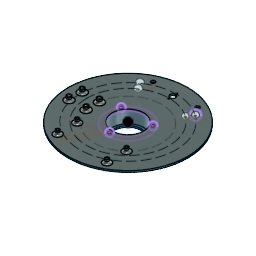
top_plate (Autodesk Fusion 360 design; units mm, degrees)
Autodesk Fusion 360 part; units mm, degrees
note: some values were not read from the file. Chosen so that the rebuilt part matches the saved one: which face or edge a step refers to. Set by a fixed rule: which sketch regions a step uses.
sketch "Sketch1" plane through (0, 0, 0) normal (0, 0, 1) x (1, 0, 0)
  circle A0 centre (0, 0) radius 80
  dimension "d1" = 160
  constraint coincident A0.centre origin
  measures "d1" diameter of A0
extrude "Extrude1" add sketch "Sketch1" along normal blind 2
sketch "Sketch4" plane through (0, 0, 2) normal (0, 0, 1) x (-1, 0, 0)
  circle A0 centre (0, 0) radius 80
  circle A1 centre (0, 0) radius 18
  dimension "d9" = 36
  constraint concentric A0 A1
  measures "d9" diameter of A1
extrude "Extrude3" cut sketch "Sketch4" against normal blind 20 contours A1 picked at (-10.335126, 0.653415)
sketch "Sketch5" plane through (0, 0, 2) normal (0, 0, 1) x (-1, 0, 0)
  circle A0 centre (0, 0) radius 18
  circle A1 centre (0, 0) radius 80
  circle A2 centre (0, 0) radius 21
  circle A3 centre (0, 0) radius 28
  dimension "d12" = 42
  dimension "d13" = 56
  constraint coincident A0.centre A1.centre
  constraint concentric A2 A3
  measures "d12" diameter of A2
  measures "d13" diameter of A3
extrude "Extrude4" add sketch "Sketch5" against normal blind 19 contours A3 picked at (25.562421, -1.391061)
sketch "Sketch6" plane through (0, 0, 2) normal (0, 0, -1) x (-1, 0, 0)
  circle A0 centre (0, 0) radius 21
  circle A1 centre (0, 0) radius 28
  circle A2 centre (0, -24.5) radius 2.15
  circle A3 centre (0, 0) radius 80
  circle A4 centre (0, 0) radius 18
  dimension "d118" = 4.3
  dimension "d119" = 24.5
  constraint vertical A0.centre A2.centre
  measures "d118" diameter of A2
  measures "d119" distance of A0.centre A2.centre
extrude "Extrude5" cut sketch "Sketch6" along normal blind 6.3 contours A2 picked at (0.840738, -23.965006)
pattern_circular "C-Pattern2" count 3 over 360 about axis through (0, 0, 2) along (0, 0, -1) of "Extrude5"
sketch "Sketch7" plane through (0, 0, 0) normal (0, 0, -1) x (1, 0, 0)
  circle A0 centre (0, 0) radius 18
  circle A1 centre (0, 0) radius 80
  circle A2 centre (0, 0) radius 45 construction
  circle A3 centre (0, 0) radius 21
  circle A4 centre (0, 0) radius 28
  dimension "d21" = 90
  constraint concentric A0 A2
  measures "d21" diameter of A2
sketch "Sketch8" plane through (0, 0, 0) normal (0, 0, -1) x (1, 0, 0)
  circle A0 centre (0, -60) radius 3.5
  circle A1 centre (0, -65.500001) radius 1
  circle A2 centre (0, -54.500001) radius 1
  dimension "d22" = 7
  dimension "d23" = 2
  dimension "d24" = 2
  measures "d22" diameter of A0
  measures "d23" diameter of A1
  measures "d24" diameter of A2
extrude "Extrude6" cut sketch "Sketch8" against normal blind 2
move_face "OffsetFaces1" offset -0.2 1 faces at (-20.895646, 2.090925, -5.666667)
ref_plane "WorkPlane1" through (0, 0, 12.125) normal (-0.819152, 0.573576, 0) x (0, 0, 1)
ref_plane "WorkPlane2" through (0, 0, 12.125) normal (-0.819152, -0.573576, 0) x (0, 0, 1)
sketch "Sketch9" plane through (0, 0, 2) normal (0, 0, 1) x (-1, 0, 0)
  circle A0 centre (0, 0) radius 80
  circle A1 centre (0, 0) radius 55 construction
  circle A2 centre (0, 0) radius 64.5 construction
  circle A3 centre (-21.217622, -12.25) radius 2.15
  circle A4 centre (21.217622, -12.25) radius 2.15
  circle A5 centre (0, 24.5) radius 2.15
  dimension "d31" = 110
  dimension "d32" = 129
  constraint coincident A0.centre A1.centre
  constraint concentric A0 A2
  measures "d31" diameter of A1
  measures "d32" diameter of A2
sketch "Sketch10" plane through (0, 0, 0) normal (-0.819152, -0.573576, 0) x (0, 0, 1)
  line L0 (2, 55.000001) -> (2, 64.500001) construction
  line L1 (2, 64.500001) -> (2, 65.000001)
  dimension "d34" = 9.5
  dimension "d43" = 0.5
  constraint vertical L0
  constraint parallel L0 L1
sketch "Sketch11" plane through (0, 0, 0) normal (-0.819152, 0.573576, 0) x (0, 0, 1)
  line L0 (2, 55.000001) -> (2, 64.500001) construction
  line L1 (2, 64.500001) -> (2, 65.000001) construction
  dimension "d36" = 9.5
  constraint vertical L0
  constraint parallel L0 L1
sketch "Sketch12" plane through (0, 0, 2) normal (0, 0, 1) x (-1, 0, 0)
  circle A0 centre (-36.995681, -52.835307) radius 1.25
  circle A1 centre (-31.546704, -45.053363) radius 1.25
  circle A2 centre (31.546704, -45.053363) radius 1.25
  circle A3 centre (36.995681, -52.835307) radius 1.25
  point P0 (-36.995681, -52.835307)
  point P1 (-31.546704, -45.053363)
  point P2 (31.546704, -45.053363)
  point P3 (36.995681, -52.835307)
  dimension "d37" = 2.5
  dimension "d38" = 2.5
  dimension "d39" = 2.5
  dimension "d40" = 2.5
  measures "d37" diameter of A0
  measures "d38" diameter of A1
  measures "d39" diameter of A2
  measures "d40" diameter of A3
extrude "Extrude7" cut sketch "Sketch12" against normal blind 2
sketch "Sketch13" plane through (0, 0, 2) normal (0, 0, 1) x (-1, 0, 0)
  circle A0 centre (37.282469, -53.244883) radius 1.25
  point P0 (37.282469, -53.244883)
  dimension "d44" = 2.5
  measures "d44" diameter of A0
sketch "Sketch14" plane through (0, 0, 2) normal (0, 0, 1) x (-1, 0, 0)
  point P0 (-37.282469, -53.244884)
sketch "Sketch15" plane through (0, 0, 2) normal (0, 0, 1) x (-1, 0, 0)
  line L0 (-38.019621, -52.118337) -> (-38.306409, -52.527913)
  circle A0 centre (-37.282469, -53.244884) radius 1.25
  circle A1 centre (-36.995681, -52.835307) radius 1.25
  line L1 (-35.971741, -53.552278) -> (-36.258529, -53.961854)
  circle A2 centre (-31.546704, -45.053363) radius 1.25
  circle A3 centre (31.546704, -45.053363) radius 1.25
  circle A4 centre (-36.995681, -52.835307) radius 1.25
  circle A5 centre (36.995681, -52.835307) radius 1.25
  circle A6 centre (0, -60) radius 3.5
  circle A7 centre (0, -65.500001) radius 1
  circle A8 centre (0, -54.500001) radius 1
  circle A9 centre (0, 0) radius 80
  circle A10 centre (0, 0) radius 18
  circle A11 centre (-21.217622, -12.25) radius 2.15
  circle A12 centre (21.217622, -12.25) radius 2.15
  circle A13 centre (0, 24.5) radius 2.15
  point P0 (-36.995681, -52.835307)
  constraint tangent L0 A0
  constraint tangent A1 L1
extrude "Extrude8" cut sketch "Sketch15" against normal blind 2 contours L0 A0 A1 A4 | A0 A1 A4 | A0 A1 L1 A4 picked at (-38.149978, -52.332254) picked at (-38.022597, -54.03365) picked at (-36.128172, -53.747937)
sketch "Sketch16" plane through (0, 0, 2) normal (0, 0, 1) x (-1, 0, 0)
  line L0 (36.258529, -53.961854) -> (35.971741, -53.552278)
  line L1 (31.546704, -45.053363) -> (36.995681, -52.835307)
  circle A0 centre (37.282469, -53.244883) radius 1.25
  circle A1 centre (36.995681, -52.835307) radius 1.25
  line L2 (38.306409, -52.527913) -> (38.019621, -52.118337)
  constraint parallel L0 L1
  constraint tangent L0 A0
  constraint parallel L1 L2
  constraint tangent A1 L2
extrude "Extrude9" cut sketch "Sketch16" sketch "Sketch13" against normal blind 2 contours L0 A0 A1 | A0 A1 L2 picked at (36.128172, -53.747937) picked at (38.149978, -52.332254) of sketch 2
move_face "OffsetFaces3" offset 0.4 1 faces at (-21.173647, 1.056733, -11.333333)
move_face "OffsetFaces4" offset -0.3 1 faces at (-17.910554, 1.792221, 0.666667)
move_face "OffsetFaces5" offset -0.2 1 faces at (3.482608, 60.348487, 0.666667)
move_face "OffsetFaces8" offset -0.15 10 faces at (-32.69855, 44.56782, 0.666667) (-35.905441, 53.446764, 0.666667) (-36.067337, 53.688803, 0.666667) (-35.905441, 53.446764, 0.666667) (-38.115217, 52.254862, 0.666667) (32.224887, 46.103395, 0.666667) (37.98261, 52.068189, 0.666667) (36.162933, 53.825329, 0.666667) (38.372708, 52.633427, 0.666667) (38.210813, 52.391388, 0.666667)
move_face "OffsetFaces9" offset -0.15 2 faces at (-0.921476, 54.888436, 1.333333) (-0.980172, 65.301855, 1.333333)
sketch "Sketch17" plane through (0, 0, 2) normal (0, 0, 1) x (-1, 0, 0)
  line L0 (0, 35.000001) -> (0, 61.150001) construction
  line L1 (0, 35.000001) -> (-33.075, 35.000001) construction
  line L2 (0, 35.000001) -> (33.075, 35.000001) construction
  line L3 (0, 61.150001) -> (-33.075, 61.150001) construction
  line L4 (0, 61.150001) -> (33.075, 61.150001) construction
  circle A0 centre (33.075, 35.000001) radius 2.5
  circle A1 centre (-33.075, 35.000001) radius 2.5
  circle A2 centre (33.075, 61.150001) radius 2.5
  circle A3 centre (-33.075, 61.150001) radius 2.5
  dimension "d59" = 26.15
  dimension "d60" = 33.075
  dimension "d61" = 33.075
  dimension "d62" = 33.075
  dimension "d63" = 33.075
  dimension "d64" = 5
  dimension "d65" = 5
  dimension "d66" = 5
  dimension "d67" = 5
  constraint vertical L0
  constraint perpendicular L0 L1
  constraint perpendicular L0 L2
  constraint perpendicular L0 L3
  constraint perpendicular L0 L4
  measures "d64" diameter of A0
  measures "d65" diameter of A1
  measures "d66" diameter of A2
  measures "d67" diameter of A3
extrude "Extrude11" add sketch "Sketch17" along normal blind 5
fillet "Fillet1" radius 3 4 edges at (-30.744182, -62.054039, 2) (-30.744182, -35.904039, 2) (35.405818, -35.904039, 2) (35.405818, -62.054039, 2)
sketch "Sketch18" plane through (0, 0, 7) normal (0, 0, 1) x (-1, 0, 0)
  circle A0 centre (33.075, 35.000001) radius 2.5
  circle A1 centre (33.075, 35.000001) radius 1.55
  dimension "d73" = 3.1
  constraint concentric A0 A1
  measures "d73" diameter of A1
sketch "Sketch19" plane through (0, 0, 7) normal (0, 0, 1) x (-1, 0, 0)
  circle A0 centre (33.075, 61.150001) radius 2.5
  circle A1 centre (33.075, 61.150001) radius 1.55
  dimension "d74" = 3.1
  constraint concentric A0 A1
  measures "d74" diameter of A1
sketch "Sketch20" plane through (0, 0, 7) normal (0, 0, 1) x (-1, 0, 0)
  circle A0 centre (-33.075, 61.150001) radius 2.5
  circle A1 centre (-33.075, 61.150001) radius 1.55
  dimension "d75" = 3.1
  constraint concentric A0 A1
  measures "d75" diameter of A1
sketch "Sketch21" plane through (0, 0, 7) normal (0, 0, 1) x (-1, 0, 0)
  circle A0 centre (-33.075, 35.000001) radius 2.5
  circle A1 centre (-33.075, 35.000001) radius 1.55
  dimension "d76" = 3.1
  constraint concentric A0 A1
  measures "d76" diameter of A1
extrude "Extrude12" cut sketch "Sketch20" sketch "Sketch19" sketch "Sketch18" sketch "Sketch21" against normal blind 5 contours A1 picked at (-33.54352, 60.507529) of sketch 2 contours A1 picked at (33.507661, 61.518054) of sketch 3 contours A1 picked at (32.61527, 34.852832) of sketch 4 contours A1 picked at (-33.54352, 34.357529)
sketch "Sketch22" plane through (0, 0, 2) normal (0, 0, 1) x (-1, 0, 0)
  line L0 (42.000001, 0) -> (64.860001, 0) construction
  line L1 (42.000001, 0) -> (42.000001, 14.113) construction
  line L2 (64.860001, 0) -> (64.860001, 14.113) construction
  line L3 (42.000001, 0) -> (42.000001, -3.667) construction
  line L4 (64.860001, 0) -> (64.860001, -3.667) construction
  circle A0 centre (64.860001, -3.667) radius 3
  circle A1 centre (64.860001, 14.113) radius 3
  circle A2 centre (42.000001, -3.667) radius 3
  circle A3 centre (42.000001, 14.113) radius 3
  dimension "d79" = 22.86
  dimension "d80" = 14.113
  dimension "d81" = 14.113
  dimension "d82" = 3.667
  dimension "d83" = 3.667
  dimension "d84" = 6
  dimension "d85" = 6
  dimension "d86" = 6
  dimension "d87" = 6
  constraint horizontal L0
  constraint perpendicular L0 L1
  constraint perpendicular L0 L2
  constraint perpendicular L0 L3
  constraint perpendicular L0 L4
  measures "d84" diameter of A0
  measures "d85" diameter of A1
  measures "d86" diameter of A2
  measures "d87" diameter of A3
extrude "Extrude13" add sketch "Sketch22" along normal blind 5
fillet "Fillet2" radius 3 4 edges at (-62.063019, -15.197846, 2) (-39.203019, -15.197846, 2) (-39.203019, 2.582154, 2) (-62.063019, 2.582154, 2)
sketch "Sketch23" plane through (0, 0, 7) normal (0, 0, 1) x (-1, 0, 0)
  circle A0 centre (42.000001, -3.667) radius 3
  circle A1 centre (42.000001, -3.667) radius 2.2
  dimension "d92" = 4.4
  constraint concentric A0 A1
  measures "d92" diameter of A1
sketch "Sketch24" plane through (0, 0, 7) normal (0, 0, 1) x (-1, 0, 0)
  circle A0 centre (42.000001, 14.113) radius 3
  circle A1 centre (42.000001, 14.113) radius 2.2
  dimension "d93" = 4.4
  constraint concentric A0 A1
  measures "d93" diameter of A1
sketch "Sketch25" plane through (0, 0, 7) normal (0, 0, 1) x (-1, 0, 0)
  circle A0 centre (64.860001, 14.113) radius 3
  circle A1 centre (64.860001, 14.113) radius 2.2
  dimension "d94" = 4.4
  constraint concentric A0 A1
  measures "d94" diameter of A1
sketch "Sketch26" plane through (0, 0, 7) normal (0, 0, 1) x (-1, 0, 0)
  circle A0 centre (64.860001, -3.667) radius 3
  circle A1 centre (64.860001, -3.667) radius 2.2
  dimension "d95" = 4.4
  constraint concentric A0 A1
  measures "d95" diameter of A1
extrude "Extrude14" cut sketch "Sketch26" sketch "Sketch25" sketch "Sketch24" sketch "Sketch23" against normal blind 5 contours A1 picked at (65.381659, -2.666178) of sketch 2 contours A1 picked at (65.381659, 15.113822) of sketch 3 contours A1 picked at (42.235337, 14.579487) of sketch 4 contours A1 picked at (41.361512, -4.296255)
sketch "Sketch27" plane through (0, 0, -17) normal (0, 0, -1) x (1, 0, 0)
  circle A0 centre (0, 0) radius 20.8
  circle A1 centre (0, 0) radius 28
  circle A2 centre (0, -24.5) radius 2.2
  circle A3 centre (-21.217623, 12.25) radius 2.2
  circle A4 centre (21.217623, 12.25) radius 2.2
sketch "Sketch28" plane through (0, 0, -17) normal (0, 0, -1) x (1, 0, 0)
  circle A0 centre (0, 0) radius 20.8
  circle A1 centre (0, 0) radius 28
  circle A2 centre (-0.389373, 0) radius 18
  dimension "d103" = 36
  measures "d103" diameter of A2
extrude "Extrude16" add sketch "Sketch28" against normal blind 2 contours A0 picked at (18.475668, -6.820428)
sketch "Sketch29" plane through (0, 0, 2) normal (0, 0, 1) x (-1, 0, 0)
sketch "Sketch30" plane through (0, 0, 2) normal (0, 0, 1) x (-1, 0, 0)
  circle A0 centre (0, 0) radius 21.075
  dimension "d106" = 42.15
  constraint coincident A0.centre origin
  measures "d106" diameter of A0
extrude "Extrude17" cut sketch "Sketch30" against normal blind 17
sketch "Sketch31" plane through (0, 0, 2) normal (0, 0, 1) x (-1, 0, 0)
  circle A0 centre (0, 0) radius 70 construction
  circle A1 centre (29.726162, -63.374721) radius 2.6
  circle A2 centre (-29.726162, -63.374721) radius 2.6
  line L0 (31.546704, -45.053363) -> (36.995681, -52.835307)
  line L1 (-31.546704, -45.053363) -> (-36.995681, -52.835307)
  dimension "d109" = 5.2
  dimension "d110" = 5.2
  dimension "d111" = 12
  dimension "d112" = 12
  dimension "d115" = 140
  constraint coincident A0.centre origin
  measures "d109" diameter of A1
  measures "d110" diameter of A2
  measures "d115" diameter of A0
extrude "Extrude18" cut sketch "Sketch31" against normal blind 3
sketch "Sketch32" plane through (0, 0, -17) normal (0, 0, -1) x (1, 0, 0)
  circle A0 centre (0, 0) radius 28
  circle A1 centre (0, 0) radius 18
  circle A2 centre (-0.389373, 0) radius 18
  dimension "d120" = 36
  measures "d120" diameter of A1
